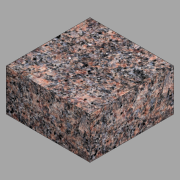
# Autodesk Inventor part: Standard - Paver
Saved by Autodesk Inventor 2022.2 (Build 262287000, 287)
## iProperties
Created: 2022-01-27
Part Number: Standard - Paver
Material: Granite, Cut, Polished
Document SubType Name: Modeling
Designer: awelt
Density: 2.7 g/cm^3
Appearance: Mahogany
Author: awelt
Autodesk Inventor part; units mm, degrees
ref_plane "YZ Plane" through (0, 0, 0) normal (1, 0, 0) x (0, 1, 0)
ref_plane "XZ Plane" through (0, 0, 0) normal (0, 1, 0) x (-1, 0, 0)
ref_plane "XY Plane" through (0, 0, 0) normal (0, 0, 1) x (1, 0, 0)
sketch "Sketch1" plane through (0, 0, 0) normal (0, 1, 0) x (-1, 0, 0)
  line L0 (0, 0) -> (-101.6, 0)
  line L1 (-101.6, 0) -> (-101.6, -101.6)
  line L2 (-101.6, -101.6) -> (0, -101.6)
  line L3 (0, -101.6) -> (0, 0)
  dimension "d0" = 101.6
  dimension "d1" = 101.6
  constraints: 8 end point, 2 parallel, 1 horizontal, 1 perpendicular
  measures "d0" distance of L2.end L1.end
  measures "d1" distance of L0.end L1.end
extrude "Extrusion1" add sketch "Sketch1" along normal blind 50.8
body "Solid1"
